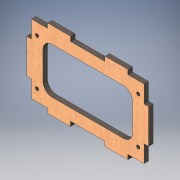
# Autodesk Inventor part: stiffenerFront
Saved by Autodesk Inventor 2019 (Build 230136000, 136)
## iProperties
Created: 2020-12-06
Part Number: stiffenerFront
Material: Дерево (береза)
Document SubType Name: Modeling
Designer: Professional
Density: 0.55 g/cm^3
Appearance: Береза — натуральный — полированный
Author: Professional
Autodesk Inventor part; units mm, degrees
ref_plane "YZ Plane" through (0, 0, 0) normal (1, 0, 0) x (0, 1, 0)
ref_plane "XZ Plane" through (0, 0, 0) normal (0, 1, 0) x (-1, 0, 0)
ref_plane "XY Plane" through (0, 0, 0) normal (0, 0, 1) x (1, 0, 0)
sketch "Эскиз1" plane through (0, 0, 0) normal (0, 0, 1) x (1, 0, 0)
  line L0 (0, 0) -> (0, 60) construction
  line L1 (0, 60) -> (-15, 60)
  line L2 (-15, 60) -> (-15, 64)
  line L3 (-15, 64) -> (-35, 64)
  line L4 (-35, 64) -> (-35, 60)
  line L5 (-35, 60) -> (-49, 60)
  line L6 (-49, 60) -> (-49, 45)
  line L7 (-49, 45) -> (-53, 45)
  line L8 (-53, 45) -> (-53, 15)
  line L9 (-53, 15) -> (-49, 15)
  line L10 (-49, 15) -> (-49, 0)
  line L11 (-49, 0) -> (-35, 0)
  line L12 (-35, 0) -> (-35, -4)
  line L13 (-35, -4) -> (-15, -4)
  line L14 (-15, -4) -> (-15, 0)
  line L15 (-15, 0) -> (0, 0)
  line L16 (0, 60) -> (15, 60)
  line L17 (15, 60) -> (15, 64)
  line L18 (15, 64) -> (35, 64)
  line L19 (35, 64) -> (35, 60)
  line L20 (35, 60) -> (49, 60)
  line L21 (49, 60) -> (49, 45)
  line L22 (49, 45) -> (53, 45)
  line L23 (53, 45) -> (53, 15)
  line L24 (53, 15) -> (49, 15)
  line L25 (49, 15) -> (49, 0)
  line L26 (49, 0) -> (35, 0)
  line L27 (35, 0) -> (35, -4)
  line L28 (35, -4) -> (15, -4)
  line L29 (15, -4) -> (15, 0)
  line L30 (15, 0) -> (0, 0)
  line L31 (-39, 50) -> (39, 50)
  line L32 (39, 50) -> (39, 10)
  line L33 (39, 10) -> (-39, 10)
  line L34 (-39, 10) -> (-39, 50)
  point P0 (-53, 30)
  point P1 (0, 30)
  point P2 (53, 30)
  dimension "d0" = 30
  dimension "d1" = 4
  dimension "d2" = 98
  dimension "d3" = 30
  dimension "d4" = 20
  dimension "d5" = 60
  dimension "d6" = 10
  dimension "d7" = 10
  dimension "d8" = 10
  constraints: 70 end point, 18 point on line, 15 symmetric about line, 13 perpendicular, 2 horizontal, 2 midpoint, 2 parallel, 1 horizontal alignment, 1 vertical, 1 other
  measures "d0" distance of L7.end L8.end
  measures "d1" distance of L11.end L12.end
  measures "d2" diameter of L10 L0
  measures "d3" diameter of L14 L0
  measures "d4" distance of L12.end L13.end
  measures "d5" distance between parallel lines of L1 L15
  measures "d6" distance between parallel lines of L31 L5
  measures "d7" distance between parallel lines of L15 L33
  measures "d8" distance between parallel lines of L10 L34
extrude "Выдавливание1" add sketch "Эскиз1" along normal blind 4
fillet "Сопряжение1" radius 8 4 edges at (-39, 10, 2) (-39, 50, 2) (39, 50, 2) (39, 10, 2)
sketch "Эскиз2" plane through (0, 0, 4) normal (0, 0, 1) x (1, 0, 0)
  line L0 (0, 0) -> (0, 60)
  line L1 (-15, 60) -> (15, 60) projected
  line L2 (-35, 60) -> (-49, 60) projected
  line L3 (-49, 0) -> (-35, 0) projected
  line L4 (-49, 60) -> (-49, 45) projected
  point P0 (44, 10)
  point P1 (44, 50)
  point P2 (-44, 10)
  point P3 (-44, 50)
  dimension "d19" = 10
  dimension "d20" = 10
  dimension "d21" = 5
  constraints: 2 end point, 2 symmetric about line, 1 midpoint, 1 vertical alignment
  measures "d19" distance from line of L2 point (-44, 50)
  measures "d20" distance from line of L3 point (-44, 10)
  measures "d21" distance from line of L4 point (-44, 50)
hole "Отверстие1" at (44, 10, 4) at (44, 50, 4) at (-44, 10, 4) at (-44, 50, 4) direction (0, 0, -1) diameter 3 end through all
